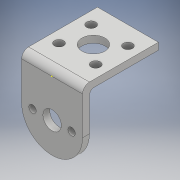
# Autodesk Inventor part: bracket motor 25GA
Saved by Autodesk Inventor 2017 (Build 210142000, 142)
## iProperties
Created: 2021-06-03
Part Number: bracket motor 25GA
Material: Generic
Document SubType Name: Modeling
Designer: ZYREX
Density: 1 g/cm^3
Appearance: Default
Author: ZYREX
Autodesk Inventor part; units mm, degrees
ref_plane "YZ Plane" through (0, 0, 0) normal (1, 0, 0) x (0, 1, 0)
ref_plane "XZ Plane" through (0, 0, 0) normal (0, 1, 0) x (-1, 0, 0)
sketch "Sketch1" plane through (0, 0, 0) normal (0, 0, 1) x (1, 0, 0)
  line L0 (-13.25, 16.5) -> (13.25, 16.5)
  line L1 (13.25, 16.5) -> (13.25, -16.5)
  line L2 (13.25, -16.5) -> (-13.25, -16.5)
  line L3 (-13.25, -16.5) -> (-13.25, 16.5)
  line L4 (-13.25, 16.5) -> (13.25, -16.5) construction
  line L5 (13.25, 16.5) -> (-13.25, -16.5) construction
  line L6 (-13.25, -16.5) -> (13.25, -16.5)
  line L7 (13.25, -16.5) -> (13.25, -13.5)
  line L8 (13.25, -13.5) -> (-13.25, -13.5)
  line L9 (-13.25, -13.5) -> (-13.25, -16.5)
  line L10 (0, 16.5) -> (0, 1.5)
  circle A0 centre (0, 1.5) radius 5
  line L11 (-8, 8.5) -> (8, -5.5) construction
  line L12 (8, 8.5) -> (-8, -5.5) construction
  circle A1 centre (8, 8.5) radius 2
  circle A2 centre (-8, 8.5) radius 2
  circle A3 centre (-8, -5.5) radius 2
  circle A4 centre (8, -5.5) radius 2
  line L13 (13.25, -13.5) -> (-13.25, -13.5)
  line L14 (-13.25, -13.5) -> (-13.25, -16.5)
  line L15 (-13.25, -16.5) -> (13.25, -16.5)
  line L16 (13.25, -16.5) -> (13.25, -13.5)
  point P0 (0, 0)
  dimension "d0" = 26.5
  dimension "d1" = 33
  dimension "d2" = 3
  dimension "d3" = 15
  dimension "d5" = 16
  dimension "d6" = 14
  dimension "d7" = 4
  dimension "d8" = 4
  dimension "d9" = 4
  dimension "d10" = 4
  constraints: 34 end point, 6 parallel, 5 centre point, 5 coincident, 5 midpoint, 3 horizontal, 3 perpendicular, 1 point on line, 1 vertical
  measures "d0" distance of L1.end L2.end
  measures "d1" distance of L0.end L1.end
  measures "d2" distance of L7.end L6.end
  measures "d3" distance of L10.start L10.end
  measures "d5" distance of L11.end L12.end
  measures "d6" distance of L12.start L11.end
  measures "d7" diameter of A1
  measures "d8" diameter of A2
  measures "d9" diameter of A3
  measures "d10" diameter of A4
extrude "Extrusion1" add sketch "Sketch1" along normal blind 3
sketch "Sketch3" plane through (0, 0, 0) normal (0, 0, 1) x (1, 0, 0)
  point P0 (0, 0)
ref_plane "Work Plane1" through (-13.25, -16.5, 1.5) normal (0, -1, 0) x (1, 0, 0)
sketch "Sketch4" plane through (-13.25, -16.5, 1.5) normal (0, -1, 0) x (1, 0, 0)
  line L0 (26.5, -1.5) -> (26.5, 1.5) projected
  line L1 (26.5, 1.5) -> (0, 1.5)
  line L2 (0, 1.5) -> (0, -18)
  line L3 (0, -18) -> (26.5, -18)
  line L4 (26.5, -18) -> (26.5, 1.5)
  arc A0 (0, -18) -> (26.5, -18) centre (13.25, -18) ccw
  point P0 (13.25, -1.5)
  dimension "d13" = 26.5
  dimension "d14" = 19.5
  constraints: 8 end point, 2 parallel, 2 point on circle, 2 tangent, 1 centre point, 1 horizontal, 1 perpendicular
  measures "d13" distance of L3.end L2.end
  measures "d14" distance of L2.end L1.end
sketch "Sketch5" plane through (-13.25, -16.5, 1.5) normal (0, -1, 0) x (1, 0, 0)
  point P0 (13.25, -1.5)
extrude "Extrusion2" add sketch "Sketch4" against normal blind 3
sketch "Sketch6" plane through (-13.25, -16.5, 1.5) normal (0, -1, 0) x (1, 0, 0)
  point P0 (13.25, -1.5)
sketch "Sketch7" plane through (-13.25, -16.5, 1.5) normal (0, -1, 0) x (1, 0, 0)
  circle A0 centre (13.25, -18) radius 4
  line L0 (26.5, -18) -> (21.75, -18)
  line L1 (21.75, -18) -> (4.75, -18)
  circle A1 centre (21.75, -18) radius 1.6
  circle A2 centre (4.75, -18) radius 1.6
  point P0 (13.25, -1.5)
  point P1 (26.5, 1.5)
  point P2 (0, -18)
  dimension "d18" = 8
  dimension "d19" = 4.75
  dimension "d20" = 17
  dimension "d21" = 3.2
  dimension "d22" = 3.2
  constraints: 4 end point, 3 centre point, 2 coincident
  measures "d18" diameter of A0
  measures "d19" distance of L0.start L0.end
  measures "d20" distance of L0.end L1.end
  measures "d21" diameter of A1
  measures "d22" diameter of A2
extrude "Extrusion3" cut sketch "Sketch7" against normal blind 3
fillet "Fillet1" radius 3 1 edges at (0, -16.5, 3)
fillet "Fillet2" radius 2 1 edges at (0, -13.5, 0)
body "Solid1"
